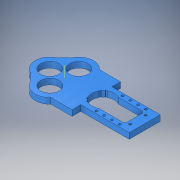
# Autodesk Inventor part: 000.401 - Опорная платформа
Saved by Autodesk Inventor 2019 (Build 230136000, 136)
## iProperties
Created: 2020-03-18
Part Number: 000.401 - Опорная платформа
Material: Пластик АБС
Document SubType Name: Modeling
Designer: Петров Иван
Density: 1.06 g/cm^3
Appearance: Голубой
Author: Петров Иван
Autodesk Inventor part; units mm, degrees
ref_plane "YZ Plane" through (0, 0, 0) normal (1, 0, 0) x (0, 1, 0)
ref_plane "XZ Plane" through (0, 0, 0) normal (0, 1, 0) x (-1, 0, 0)
ref_plane "XY Plane" through (0, 0, 0) normal (0, 0, 1) x (1, 0, 0)
sketch "Эскиз1" plane through (0, 0, 0) normal (0, 1, 0) x (-1, 0, 0)
  circle A0 centre (0, 0) radius 13.8
  circle A1 centre (-8, 0) radius 1.2
  circle A2 centre (0, -8) radius 1.2
  circle A3 centre (8, 0) radius 1.2
  circle A4 centre (0, 8) radius 1.2
  circle A5 centre (-7.7782, 7.7782) radius 1.2813
  circle A6 centre (-11, 0) radius 1.2813
  circle A7 centre (-7.7782, -7.7782) radius 1.2813
  circle A8 centre (0, -11) radius 1.2812
  circle A9 centre (7.7782, -7.7782) radius 1.2812
  circle A10 centre (11, 0) radius 1.2813
  circle A11 centre (7.7782, 7.7782) radius 1.2812
  circle A12 centre (0, 11) radius 1.2812
  circle A13 centre (0, 0) radius 5
  circle A14 centre (0, 0) radius 14
  circle A15 centre (0, 0) radius 1.55
  circle A16 centre (0, 0) radius 1.75
  circle A17 centre (0, 0) radius 25
  dimension "d0" = 50
  constraints: 18 centre point, 1 coincident
  measures "d0" diameter of A17
extrude "Выдавливание1" add sketch "Эскиз1" along normal blind 6 contours A0 | A1 | A2 | A3 | A4 | A5 | A6 | A7 | A8 | A9 | A10 | A11 | A12 | A13 | A14 | A15 | A16 | A17
sketch "Эскиз2" plane through (0, 6, 0) normal (0, 1, 0) x (1, 0, 0)
  line L0 (25, 0) -> (100, 0)
  circle A0 centre (100, 0) radius 25
  line L1 (50, 0) -> (50, -20)
  line L2 (50, 0) -> (50, 20)
  circle A1 centre (0, 0) radius 25 projected
  arc A2 (4.9455, 24.506) -> (95.0545, 24.506) centre (50, 247.5) ccw
  arc A3 (95.0545, -24.506) -> (4.9455, -24.506) centre (50, -247.5) ccw
  line L3 (100, 25) -> (0, 25)
  line L4 (0, -25) -> (100, -25)
  line L5 (50, 20) -> (50, 25)
  line L6 (50, -20) -> (50, -25)
  line L7 (50, 25) -> (50, -25)
  dimension "d3" = 100
  dimension "d4" = 50
  dimension "d5" = 20
  dimension "d6" = 20
  constraints: 16 end point, 15 point on circle, 3 centre point, 3 tangent, 2 midpoint, 2 vertical, 1 coincident, 1 collinear, 1 horizontal, 1 point on line
  measures "d3" distance of point (0, 0) L0.end
  measures "d4" diameter of A0
  measures "d5" distance of L1.start L1.end
  measures "d6" distance of L1.start L2.end
extrude "Выдавливание2" add sketch "Эскиз2" against normal blind 6 contours A1 A2 L2 L0 | L0 L1 A3 A1 | A1 L3 L5 A2 | A3 L6 L4 A1
sketch "Эскиз7" plane through (0, 6, 0) normal (0, 1, 0) x (1, 0, 0)
  line L0 (100, 0) -> (100, 15)
  line L1 (100, 0) -> (100, -15)
  circle A0 centre (100, 15) radius 3
  circle A1 centre (100, -15) radius 3
  line L2 (100, 0) -> (115, 0)
  circle A2 centre (115, 0) radius 3
  point P0 (0, 0)
  dimension "d23" = 15
  dimension "d24" = 15
  dimension "d25" = 6
  dimension "d26" = 6
  dimension "d27" = 15
  dimension "d28" = 6
  constraints: 6 end point, 3 centre point, 3 coincident, 2 vertical, 1 horizontal, 1 other
  measures "d23" distance of L0.start L0.end
  measures "d24" distance of L0.start L1.end
  measures "d25" diameter of A0
  measures "d26" diameter of A1
  measures "d27" distance of L0.start L2.end
  measures "d28" diameter of A2
extrude "Выдавливание7" [suppressed]
move faces "Перенос1" translate (33, 0, 0) faces at (50, 4, 8.3333)
sketch "Эскиз11" plane through (0, 6, 0) normal (0, 1, 0) x (1, 0, 0)
  line L0 (83, -25) -> (0, -25) projected
  line L1 (83, -25) -> (33, -25)
  line L2 (33, -25) -> (33, -16)
  line L3 (33, -16) -> (83, -16)
  line L4 (83, -16) -> (83, -25)
  point P0 (0, 0)
  dimension "d41" = 50
  dimension "d42" = 9
  constraints: 8 end point, 2 parallel, 1 horizontal, 1 perpendicular
  measures "d41" distance of L2.end L3.end
  measures "d42" distance of L1.end L2.end
extrude "Выдавливание11" cut sketch "Эскиз11" against normal blind 10
mirror "Зеркальное отражение2" about plane through (0, 0, 0) normal (0, 0, 1) of "Выдавливание11"
sketch "Эскиз12" plane through (0, 6, 0) normal (0, 1, 0) x (1, 0, 0)
  line L0 (32.95, -10) -> (71.0915, -10)
  line L1 (32.95, -10) -> (32.95, -11.4565)
  arc A0 (32.95, -11.4565) -> (33.5, -11.5) centre (33.5, -8) ccw
  line L2 (33.5, -11.5) -> (42, -11.5)
  line L3 (42, -11.5) -> (42, -13)
  line L4 (42, -13) -> (43.5, -13)
  line L5 (43.5, -13) -> (43.5, -15)
  line L6 (43.5, -15) -> (50, -15)
  line L7 (50, -15) -> (50, -13)
  line L8 (50, -13) -> (51.5, -13)
  line L9 (51.5, -13) -> (51.5, -15)
  line L10 (51.5, -15) -> (58, -15)
  line L11 (58, -15) -> (58, -13)
  line L12 (58, -13) -> (59.5, -13)
  line L13 (59.5, -13) -> (59.5, -15)
  line L14 (59.5, -15) -> (66, -15)
  line L15 (66, -15) -> (66, -13)
  line L16 (66, -13) -> (67.5, -13)
  line L17 (67.5, -13) -> (67.5, -15)
  line L18 (67.5, -15) -> (74, -15)
  line L19 (74, -15) -> (74, -13)
  line L20 (74, -13) -> (75.5, -13)
  line L21 (75.5, -13) -> (75.5, -11.25)
  line L22 (75.5, -11.25) -> (77.5, -11.25)
  line L23 (77.5, -11.25) -> (77.5, -4.75)
  line L24 (77.5, -4.75) -> (75.5, -4.75)
  line L25 (75.5, -4.75) -> (75.5, 4.75)
  line L26 (75.5, 4.75) -> (77.5, 4.75)
  line L27 (77.5, 4.75) -> (77.5, 11.25)
  line L28 (77.5, 11.25) -> (75.5, 11.25)
  line L29 (75.5, 11.25) -> (75.5, 13)
  line L30 (75.5, 13) -> (74, 13)
  line L31 (74, 13) -> (74, 15)
  line L32 (74, 15) -> (67.5, 15)
  line L33 (67.5, 15) -> (67.5, 13)
  line L34 (67.5, 13) -> (66, 13)
  line L35 (66, 13) -> (66, 15)
  line L36 (66, 15) -> (59.5, 15)
  line L37 (59.5, 15) -> (59.5, 13)
  line L38 (59.5, 13) -> (58, 13)
  line L39 (58, 13) -> (58, 15)
  line L40 (58, 15) -> (51.5, 15)
  line L41 (51.5, 15) -> (51.5, 13)
  line L42 (51.5, 13) -> (50, 13)
  line L43 (50, 13) -> (50, 15)
  line L44 (50, 15) -> (43.5, 15)
  line L45 (43.5, 15) -> (43.5, 13)
  line L46 (43.5, 13) -> (42, 13)
  line L47 (42, 13) -> (42, 11.5)
  line L48 (42, 11.5) -> (33.5, 11.5)
  arc A1 (33.5, 11.5) -> (32.9779, 11.4608) centre (33.5, 8) ccw
  line L49 (32.9779, 11.4608) -> (32.9779, 10)
  line L50 (71.0279, 10) -> (32.9779, 10)
  line L51 (71.0279, 10) -> (71.1016, 9.9543)
  arc A2 (72.4429, 8.5313) -> (71.1016, 9.9543) centre (73, 10.4) ccw
  line L52 (72.4429, 8.5313) -> (72.5, 8.4256)
  line L53 (72.5, -8.5152) -> (72.5, 8.4256)
  arc A3 (71.0915, -10) -> (72.5, -8.5152) centre (73, -10.4) ccw
  circle A4 centre (54.75, -13.5) radius 1.25
  circle A5 centre (70.75, -13.5) radius 1.25
  circle A6 centre (76, 8) radius 1.25
  circle A7 centre (70.75, 13.5) radius 1.25
  circle A8 centre (62.75, 13.5) radius 1.25
  circle A9 centre (54.75, 13.5) radius 1.25
  circle A10 centre (46.75, 13.5) radius 1.25
  circle A11 centre (76, -8) radius 1.25
  circle A12 centre (62.75, -13.5) radius 1.25
  circle A13 centre (46.75, -13.5) radius 1.25
  arc A14 (32.95, -9.25) -> (31, -7.3) centre (31, -9.25) ccw
  line L54 (32.95, -9.25) -> (32.95, -10)
  line L55 (32.95, -10) -> (48.95, -10)
  line L56 (48.95, -10) -> (48.75, -9.8)
  line L57 (48.75, -7.0711) -> (48.75, -9.8)
  arc A15 (48.75, -7.0711) -> (48.75, 7.0711) centre (40, 0) ccw
  line L58 (48.75, 9.8) -> (48.75, 7.0711)
  line L59 (48.75, 9.8) -> (48.95, 10)
  line L60 (48.95, 10) -> (32.95, 10)
  line L61 (32.95, 10) -> (32.95, 9.25)
  arc A16 (31, 7.3) -> (32.95, 9.25) centre (31, 9.25) ccw
  line L62 (31, 7.3) -> (30, 7.3)
  line L63 (30, 7.3) -> (30, -7.3)
  line L64 (30, -7.3) -> (31, -7.3)
  circle A17 centre (40, 0) radius 9.1
  line L65 (48.95, 10) -> (32.95, 10)
  line L66 (42, 13) -> (42, 11.5)
  line L67 (33.5, 13) -> (42, 13)
  line L68 (33.5, 11.5) -> (33.5, 13)
  line L69 (42, 11.5) -> (33.5, 11.5)
  arc A18 (33.5, 13) -> (32.9501, 12.9697) centre (33.5, 8) ccw
  spline S0 degree 3 poles (32.9501, 12.9697) (32.9501, 12.9689) (32.9503, 12.9605) (32.9503, 12.9597) (32.9503, 12.959) (32.9503, 12.9582) (32.9503, 12.9574) (32.9503, 12.9541) (32.9504, 12.9501) (32.9505, 12.9454) (32.9505, 12.9438) (32.9505, 12.9421) (32.9505, 12.9403) (32.9505, 12.9395) (32.9506, 12.9387) (32.9506, 12.9379) (32.9506, 12.9353) (32.9506, 12.9324) (32.9507, 12.9294) (32.9508, 12.9234) (32.9509, 12.9168) (32.951, 12.9095) (32.951, 12.9077) (32.951, 12.9059) (32.951, 12.9041) (32.9511, 12.8983) (32.9512, 12.8922) (32.9513, 12.8858) (32.9514, 12.8786) (32.9515, 12.8711) (32.9516, 12.8629) (32.9516, 12.8601) (32.9517, 12.8571) (32.9517, 12.8541) (32.9519, 12.8456) (32.952, 12.8366) (32.9521, 12.8272) (32.9523, 12.8162) (32.9524, 12.8046) (32.9526, 12.7924) (32.9528, 12.7801) (32.953, 12.7673) (32.9532, 12.7538) (32.9533, 12.7471) (32.9534, 12.7401) (32.9535, 12.7331) (32.9536, 12.7264) (32.9537, 12.7196) (32.9538, 12.7126) (32.954, 12.6978) (32.9542, 12.6823) (32.9545, 12.6664) (32.9547, 12.6528) (32.9549, 12.6387) (32.9551, 12.6244) (32.9553, 12.6118) (32.9555, 12.5991) (32.9557, 12.5862) (32.9558, 12.5798) (32.9559, 12.5734) (32.956, 12.5669) (32.9562, 12.5538) (32.9564, 12.5402) (32.9567, 12.5259) (32.957, 12.5031) (32.9574, 12.4796) (32.9578, 12.4556) (32.958, 12.4458) (32.9581, 12.4359) (32.9583, 12.4258) (32.9585, 12.4158) (32.9586, 12.4056) (32.9588, 12.3954) (32.9592, 12.3748) (32.9595, 12.354) (32.9599, 12.3329) (32.9601, 12.3203) (32.9603, 12.3076) (32.9605, 12.2948) (32.9607, 12.286) (32.9608, 12.2773) (32.961, 12.2685) (32.9614, 12.2466) (32.9618, 12.2245) (32.9622, 12.2021) (32.9624, 12.1909) (32.9626, 12.1796) (32.9628, 12.1683) (32.963, 12.1568) (32.9632, 12.1454) (32.9634, 12.1339) (32.9638, 12.1145) (32.9642, 12.0951) (32.9645, 12.0752) (32.9646, 12.0714) (32.9647, 12.0676) (32.9648, 12.0637) (32.9649, 12.0547) (32.9651, 12.0456) (32.9653, 12.0365) (32.9656, 12.0216) (32.9659, 12.0067) (32.9662, 11.9916) (32.9666, 11.9672) (32.9671, 11.9425) (32.9676, 11.9178) (32.9681, 11.8931) (32.9687, 11.8682) (32.9692, 11.8433) (32.9697, 11.8183) (32.9702, 11.7932) (32.9708, 11.7681) (32.9719, 11.7177) (32.973, 11.6669) (32.9742, 11.6157) (32.9754, 11.5645) (32.9766, 11.5128) (32.9779, 11.4608) knots 0.064201 0.064201 0.064201 0.064201 0.072529 0.072529 0.072529 0.080597 0.080597 0.080597 0.113423 0.113423 0.113423 0.125 0.125 0.125 0.12994 0.12994 0.12994 0.146482 0.146482 0.146482 0.17952 0.17952 0.17952 0.1875 0.1875 0.1875 0.212571 0.212571 0.212571 0.240274 0.240274 0.240274 0.25 0.25 0.25 0.277642 0.277642 0.277642 0.310147 0.310147 0.310147 0.342874 0.342874 0.342874 0.3593 0.3593 0.3593 0.375 0.375 0.375 0.408683 0.408683 0.408683 0.4375 0.4375 0.4375 0.462715 0.462715 0.462715 0.475013 0.475013 0.475013 0.5 0.5 0.5 0.540067 0.540067 0.540067 0.556372 0.556372 0.556372 0.572723 0.572723 0.572723 0.605497 0.605497 0.605497 0.625 0.625 0.625 0.638264 0.638264 0.638264 0.671081 0.671081 0.671081 0.6875 0.6875 0.6875 0.704131 0.704131 0.704131 0.732078 0.732078 0.732078 0.737463 0.737463 0.737463 0.75 0.75 0.75 0.770238 0.770238 0.770238 0.802948 0.802948 0.802948 0.835688 0.835688 0.835688 0.868461 0.868461 0.868461 0.93413 0.93413 0.93413 1 1 1 1
  arc A19 (33.5, 11.5) -> (32.9779, 11.4608) centre (33.5, 8) ccw
  line L70 (33.5, 11.5) -> (33.5, 13)
  arc A20 (32.9501, 12.9697) -> (28.5, 8) centre (33.5, 8) ccw
  line L71 (28.5, 7.3) -> (28.5, 8)
  line L72 (28.5, -7.3) -> (28.5, 7.3)
  line L73 (28.5, -8) -> (28.5, -7.3)
  arc A21 (28.5, -8) -> (32.9271, -12.9671) centre (33.5, -8) ccw
  line L74 (42, -13) -> (33.5, -13)
  arc A22 (32.9271, -12.9671) -> (33.5, -13) centre (33.5, -8) ccw
  line L75 (43.5, -16) -> (43.5, -15)
  line L76 (50, -16) -> (43.5, -16)
  line L77 (50, -15) -> (50, -16)
  line L78 (43.5, -15) -> (50, -15)
  line L79 (51.5, -16) -> (51.5, -15)
  line L80 (58, -16) -> (51.5, -16)
  line L81 (58, -15) -> (58, -16)
  line L82 (51.5, -15) -> (58, -15)
  line L83 (59.5, -16) -> (59.5, -15)
  line L84 (66, -16) -> (59.5, -16)
  line L85 (66, -15) -> (66, -16)
  line L86 (59.5, -15) -> (66, -15)
  line L87 (67.5, -16) -> (67.5, -15)
  line L88 (74, -16) -> (67.5, -16)
  line L89 (74, -15) -> (74, -16)
  line L90 (67.5, -15) -> (74, -15)
  line L91 (78.5, -11.25) -> (77.5, -11.25)
  line L92 (78.5, -4.75) -> (78.5, -11.25)
  line L93 (77.5, -4.75) -> (78.5, -4.75)
  line L94 (77.5, -11.25) -> (77.5, -4.75)
  line L95 (78.5, 4.75) -> (77.5, 4.75)
  line L96 (78.5, 11.25) -> (78.5, 4.75)
  line L97 (77.5, 11.25) -> (78.5, 11.25)
  line L98 (77.5, 4.75) -> (77.5, 11.25)
  line L99 (74, 16) -> (74, 15)
  line L100 (67.5, 16) -> (74, 16)
  line L101 (67.5, 15) -> (67.5, 16)
  line L102 (74, 15) -> (67.5, 15)
  line L103 (66, 16) -> (66, 15)
  line L104 (59.5, 16) -> (66, 16)
  line L105 (59.5, 15) -> (59.5, 16)
  line L106 (66, 15) -> (59.5, 15)
  line L107 (51.5, 16) -> (58, 16)
  line L108 (58, 16) -> (58, 15)
  line L109 (51.5, 16) -> (58, 16)
  line L110 (51.5, 15) -> (51.5, 16)
  line L111 (58, 15) -> (51.5, 15)
  line L112 (50, 16) -> (50, 15)
  line L113 (43.5, 16) -> (50, 16)
  line L114 (43.5, 15) -> (43.5, 16)
  line L115 (50, 15) -> (43.5, 15)
  spline S1 degree 3 poles (32.95, -11.4565) (32.9497, -11.4689) (32.9495, -11.4813) (32.9492, -11.4937) (32.9487, -11.5195) (32.9482, -11.5454) (32.9477, -11.5712) (32.9472, -11.5969) (32.9467, -11.6225) (32.9462, -11.6481) (32.9456, -11.6821) (32.9449, -11.716) (32.9443, -11.7496) (32.944, -11.7664) (32.9437, -11.7832) (32.9434, -11.7999) (32.943, -11.825) (32.9425, -11.85) (32.9421, -11.8749) (32.942, -11.8808) (32.9419, -11.8868) (32.9418, -11.8927) (32.9415, -11.9115) (32.9412, -11.9304) (32.9409, -11.9492) (32.9407, -11.9616) (32.9405, -11.9739) (32.9403, -11.986) (32.9401, -11.9983) (32.9399, -12.0104) (32.9397, -12.0224) (32.9396, -12.0258) (32.9396, -12.0292) (32.9395, -12.0327) (32.9392, -12.0531) (32.9389, -12.0734) (32.9386, -12.0936) (32.9379, -12.1324) (32.9374, -12.1706) (32.9368, -12.208) (32.9367, -12.2155) (32.9366, -12.2229) (32.9365, -12.2303) (32.9362, -12.2507) (32.9359, -12.2709) (32.9356, -12.2908) (32.9353, -12.3141) (32.935, -12.3369) (32.9346, -12.3594) (32.9345, -12.3699) (32.9343, -12.3802) (32.9342, -12.3905) (32.9341, -12.3973) (32.934, -12.4041) (32.9339, -12.4108) (32.9339, -12.4142) (32.9338, -12.4176) (32.9338, -12.421) (32.9336, -12.4356) (32.9334, -12.4501) (32.9332, -12.4643) (32.9331, -12.4696) (32.9331, -12.4747) (32.933, -12.4799) (32.9328, -12.4947) (32.9326, -12.509) (32.9324, -12.5227) (32.9324, -12.527) (32.9323, -12.5314) (32.9323, -12.5357) (32.932, -12.5537) (32.9318, -12.5714) (32.9316, -12.5885) (32.9314, -12.6056) (32.9312, -12.6223) (32.931, -12.6384) (32.9308, -12.6545) (32.9306, -12.6702) (32.9304, -12.6853) (32.9303, -12.6935) (32.9302, -12.7016) (32.9301, -12.7095) (32.93, -12.7161) (32.9299, -12.7227) (32.9298, -12.7291) (32.9298, -12.7362) (32.9297, -12.7431) (32.9296, -12.7499) (32.9295, -12.7567) (32.9294, -12.7633) (32.9293, -12.7697) (32.9293, -12.7755) (32.9292, -12.7811) (32.9291, -12.7866) (32.9291, -12.7934) (32.929, -12.8001) (32.9289, -12.8066) (32.9288, -12.8161) (32.9287, -12.8252) (32.9286, -12.8338) (32.9286, -12.8358) (32.9286, -12.8378) (32.9285, -12.8397) (32.9285, -12.8437) (32.9284, -12.8476) (32.9284, -12.8514) (32.9282, -12.8675) (32.928, -12.8819) (32.9279, -12.8948) (32.9278, -12.9027) (32.9277, -12.9101) (32.9276, -12.9167) (32.9276, -12.9234) (32.9275, -12.9295) (32.9274, -12.9349) (32.9274, -12.9403) (32.9273, -12.945) (32.9273, -12.949) (32.9272, -12.953) (32.9272, -12.9564) (32.9272, -12.9591) (32.9271, -12.9644) (32.9271, -12.9671) (32.9271, -12.9671) knots 0 0 0 0 0.015717 0.015717 0.015717 0.048574 0.048574 0.048574 0.081322 0.081322 0.081322 0.125 0.125 0.125 0.146869 0.146869 0.146869 0.179663 0.179663 0.179663 0.1875 0.1875 0.1875 0.212348 0.212348 0.212348 0.228682 0.228682 0.228682 0.245216 0.245216 0.245216 0.25 0.25 0.25 0.278672 0.278672 0.278672 0.333784 0.333784 0.333784 0.344755 0.344755 0.344755 0.375 0.375 0.375 0.410279 0.410279 0.410279 0.42665 0.42665 0.42665 0.4375 0.4375 0.4375 0.443003 0.443003 0.443003 0.466515 0.466515 0.466515 0.475131 0.475131 0.475131 0.5 0.5 0.5 0.507943 0.507943 0.507943 0.541148 0.541148 0.541148 0.574177 0.574177 0.574177 0.607119 0.607119 0.607119 0.625 0.625 0.625 0.640065 0.640065 0.640065 0.65654 0.65654 0.65654 0.672965 0.672965 0.672965 0.6875 0.6875 0.6875 0.705429 0.705429 0.705429 0.731487 0.731487 0.731487 0.737562 0.737562 0.737562 0.75 0.75 0.75 0.803346 0.803346 0.803346 0.83629 0.83629 0.83629 0.869201 0.869201 0.869201 0.902051 0.902051 0.902051 0.934818 0.934818 0.934818 1 1 1 1
  line L116 (32.75, -12.7684) -> (32.75, -11.4565)
  line L117 (32.75, -11.4565) -> (32.75, -10)
  line L118 (32.95, -10) -> (32.75, -10)
  line L119 (32.95, -11.4565) -> (32.75, -11.4565)
  line L120 (32.75, -12.7684) -> (32.75, -11.4565)
  line L121 (32.9271, -12.9671) -> (32.75, -12.7684)
  spline S2 degree 3 poles (32.95, -11.4565) (32.9497, -11.4689) (32.9495, -11.4813) (32.9492, -11.4937) (32.9487, -11.5195) (32.9482, -11.5454) (32.9477, -11.5712) (32.9472, -11.5969) (32.9467, -11.6225) (32.9462, -11.6481) (32.9456, -11.6821) (32.9449, -11.716) (32.9443, -11.7496) (32.944, -11.7664) (32.9437, -11.7832) (32.9434, -11.7999) (32.943, -11.825) (32.9425, -11.85) (32.9421, -11.8749) (32.942, -11.8808) (32.9419, -11.8868) (32.9418, -11.8927) (32.9415, -11.9115) (32.9412, -11.9304) (32.9409, -11.9492) (32.9407, -11.9616) (32.9405, -11.9739) (32.9403, -11.986) (32.9401, -11.9983) (32.9399, -12.0104) (32.9397, -12.0224) (32.9396, -12.0258) (32.9396, -12.0292) (32.9395, -12.0327) (32.9392, -12.0531) (32.9389, -12.0734) (32.9386, -12.0936) (32.938, -12.1324) (32.9374, -12.1706) (32.9368, -12.208) (32.9367, -12.2155) (32.9366, -12.2229) (32.9365, -12.2303) (32.9362, -12.2507) (32.9359, -12.2709) (32.9356, -12.2908) (32.9353, -12.3141) (32.935, -12.3369) (32.9346, -12.3594) (32.9345, -12.3699) (32.9344, -12.3802) (32.9342, -12.3905) (32.9341, -12.3973) (32.934, -12.4041) (32.9339, -12.4108) (32.9339, -12.4142) (32.9338, -12.4176) (32.9338, -12.421) (32.9336, -12.4356) (32.9334, -12.4501) (32.9332, -12.4643) (32.9331, -12.4696) (32.9331, -12.4747) (32.933, -12.4799) (32.9328, -12.4947) (32.9326, -12.509) (32.9324, -12.5227) (32.9324, -12.527) (32.9323, -12.5314) (32.9323, -12.5357) (32.932, -12.5537) (32.9318, -12.5714) (32.9316, -12.5885) (32.9314, -12.6056) (32.9312, -12.6223) (32.931, -12.6384) (32.9308, -12.6545) (32.9306, -12.6702) (32.9304, -12.6853) (32.9303, -12.6935) (32.9302, -12.7016) (32.9301, -12.7095) (32.93, -12.7161) (32.9299, -12.7227) (32.9298, -12.7291) (32.9298, -12.7362) (32.9297, -12.7431) (32.9296, -12.7499) (32.9295, -12.7567) (32.9294, -12.7633) (32.9294, -12.7697) (32.9293, -12.7755) (32.9292, -12.7811) (32.9292, -12.7866) (32.9291, -12.7934) (32.929, -12.8001) (32.9289, -12.8066) (32.9288, -12.8161) (32.9287, -12.8252) (32.9286, -12.8338) (32.9286, -12.8358) (32.9286, -12.8378) (32.9285, -12.8397) (32.9285, -12.8437) (32.9284, -12.8476) (32.9284, -12.8514) (32.9282, -12.8675) (32.928, -12.8819) (32.9279, -12.8948) (32.9278, -12.9027) (32.9277, -12.9101) (32.9277, -12.9167) (32.9276, -12.9234) (32.9275, -12.9295) (32.9274, -12.9349) (32.9274, -12.9403) (32.9273, -12.945) (32.9273, -12.949) (32.9272, -12.953) (32.9272, -12.9564) (32.9272, -12.9591) (32.9271, -12.9644) (32.9271, -12.9671) (32.9271, -12.9671) knots 0 0 0 0 0.015717 0.015717 0.015717 0.048574 0.048574 0.048574 0.081322 0.081322 0.081322 0.125 0.125 0.125 0.146869 0.146869 0.146869 0.179663 0.179663 0.179663 0.1875 0.1875 0.1875 0.212348 0.212348 0.212348 0.228682 0.228682 0.228682 0.245216 0.245216 0.245216 0.25 0.25 0.25 0.278672 0.278672 0.278672 0.333784 0.333784 0.333784 0.344755 0.344755 0.344755 0.375 0.375 0.375 0.410279 0.410279 0.410279 0.42665 0.42665 0.42665 0.4375 0.4375 0.4375 0.443003 0.443003 0.443003 0.466515 0.466515 0.466515 0.475131 0.475131 0.475131 0.5 0.5 0.5 0.507943 0.507943 0.507943 0.541148 0.541148 0.541148 0.574177 0.574177 0.574177 0.607119 0.607119 0.607119 0.625 0.625 0.625 0.640065 0.640065 0.640065 0.65654 0.65654 0.65654 0.672965 0.672965 0.672965 0.6875 0.6875 0.6875 0.705429 0.705429 0.705429 0.731487 0.731487 0.731487 0.737562 0.737562 0.737562 0.75 0.75 0.75 0.803346 0.803346 0.803346 0.83629 0.83629 0.83629 0.869201 0.869201 0.869201 0.902051 0.902051 0.902051 0.934818 0.934818 0.934818 1 1 1 1
  line L122 (32.75, -10) -> (32.95, -10)
  line L123 (32.75, -11.4565) -> (32.75, -10)
  line L124 (32.95, -11.4565) -> (32.75, -11.4565)
  line L125 (32.95, -10) -> (32.95, -11.4565)
  line L126 (32.75, 11.4608) -> (32.9779, 11.4608)
  spline S3 degree 3 poles (32.9501, 12.9697) (32.9501, 12.9689) (32.9503, 12.9605) (32.9503, 12.9597) (32.9503, 12.959) (32.9503, 12.9582) (32.9503, 12.9574) (32.9503, 12.9541) (32.9504, 12.9501) (32.9505, 12.9454) (32.9505, 12.9438) (32.9505, 12.9421) (32.9505, 12.9403) (32.9505, 12.9395) (32.9506, 12.9387) (32.9506, 12.9379) (32.9506, 12.9353) (32.9506, 12.9324) (32.9507, 12.9294) (32.9508, 12.9234) (32.9509, 12.9168) (32.951, 12.9095) (32.951, 12.9077) (32.951, 12.9059) (32.951, 12.9041) (32.9511, 12.8983) (32.9512, 12.8922) (32.9513, 12.8858) (32.9514, 12.8786) (32.9515, 12.8711) (32.9516, 12.8629) (32.9516, 12.8601) (32.9517, 12.8571) (32.9517, 12.8541) (32.9519, 12.8456) (32.952, 12.8366) (32.9521, 12.8272) (32.9523, 12.8162) (32.9524, 12.8046) (32.9526, 12.7924) (32.9528, 12.7801) (32.953, 12.7673) (32.9532, 12.7538) (32.9533, 12.7471) (32.9534, 12.7401) (32.9535, 12.7331) (32.9536, 12.7264) (32.9537, 12.7196) (32.9538, 12.7126) (32.954, 12.6978) (32.9542, 12.6823) (32.9545, 12.6664) (32.9547, 12.6528) (32.9549, 12.6387) (32.9551, 12.6244) (32.9553, 12.6118) (32.9555, 12.5991) (32.9557, 12.5862) (32.9558, 12.5798) (32.9559, 12.5734) (32.956, 12.5669) (32.9562, 12.5538) (32.9564, 12.5402) (32.9567, 12.5259) (32.957, 12.5031) (32.9574, 12.4796) (32.9578, 12.4556) (32.958, 12.4458) (32.9581, 12.4359) (32.9583, 12.4258) (32.9585, 12.4158) (32.9586, 12.4056) (32.9588, 12.3954) (32.9591, 12.3748) (32.9595, 12.354) (32.9599, 12.3329) (32.9601, 12.3203) (32.9603, 12.3076) (32.9605, 12.2948) (32.9607, 12.286) (32.9608, 12.2773) (32.961, 12.2685) (32.9614, 12.2466) (32.9618, 12.2245) (32.9622, 12.2021) (32.9624, 12.1909) (32.9626, 12.1796) (32.9628, 12.1683) (32.963, 12.1568) (32.9632, 12.1454) (32.9634, 12.1339) (32.9638, 12.1145) (32.9642, 12.0951) (32.9645, 12.0752) (32.9646, 12.0714) (32.9647, 12.0676) (32.9648, 12.0637) (32.9649, 12.0547) (32.9651, 12.0456) (32.9653, 12.0365) (32.9656, 12.0216) (32.9659, 12.0067) (32.9662, 11.9916) (32.9666, 11.9672) (32.9671, 11.9425) (32.9676, 11.9178) (32.9681, 11.8931) (32.9686, 11.8682) (32.9692, 11.8433) (32.9697, 11.8183) (32.9702, 11.7932) (32.9708, 11.7681) (32.9719, 11.7177) (32.973, 11.6669) (32.9742, 11.6157) (32.9754, 11.5645) (32.9766, 11.5128) (32.9779, 11.4608) knots 0.064201 0.064201 0.064201 0.064201 0.072529 0.072529 0.072529 0.080597 0.080597 0.080597 0.113423 0.113423 0.113423 0.125 0.125 0.125 0.12994 0.12994 0.12994 0.146482 0.146482 0.146482 0.17952 0.17952 0.17952 0.1875 0.1875 0.1875 0.212571 0.212571 0.212571 0.240274 0.240274 0.240274 0.25 0.25 0.25 0.277642 0.277642 0.277642 0.310147 0.310147 0.310147 0.342874 0.342874 0.342874 0.3593 0.3593 0.3593 0.375 0.375 0.375 0.408683 0.408683 0.408683 0.4375 0.4375 0.4375 0.462715 0.462715 0.462715 0.475013 0.475013 0.475013 0.5 0.5 0.5 0.540067 0.540067 0.540067 0.556372 0.556372 0.556372 0.572723 0.572723 0.572723 0.605497 0.605497 0.605497 0.625 0.625 0.625 0.638264 0.638264 0.638264 0.671081 0.671081 0.671081 0.6875 0.6875 0.6875 0.704131 0.704131 0.704131 0.732078 0.732078 0.732078 0.737463 0.737463 0.737463 0.75 0.75 0.75 0.770238 0.770238 0.770238 0.802948 0.802948 0.802948 0.835688 0.835688 0.835688 0.868461 0.868461 0.868461 0.93413 0.93413 0.93413 1 1 1 1
  line L127 (32.7706, 12.7443) -> (32.9501, 12.9697)
  line L128 (32.75, 12.7184) -> (32.7706, 12.7443)
  line L129 (32.75, 11.4608) -> (32.75, 12.7184)
  line L130 (32.9779, 10) -> (32.75, 10)
  line L131 (32.9779, 11.4608) -> (32.9779, 10)
  line L132 (32.75, 11.4608) -> (32.9779, 11.4608)
  line L133 (32.75, 10) -> (32.75, 11.4608)
  arc A23 (32.95, -11.4565) -> (33.5, -11.5) centre (33.5, -8) ccw
  spline S4 degree 3 poles (32.95, -11.4565) (32.9497, -11.4689) (32.9495, -11.4813) (32.9492, -11.4937) (32.9487, -11.5195) (32.9482, -11.5454) (32.9477, -11.5712) (32.9472, -11.5969) (32.9467, -11.6225) (32.9462, -11.6481) (32.9456, -11.6821) (32.9449, -11.716) (32.9443, -11.7496) (32.944, -11.7664) (32.9437, -11.7832) (32.9434, -11.7999) (32.943, -11.825) (32.9425, -11.85) (32.9421, -11.8749) (32.942, -11.8808) (32.9419, -11.8868) (32.9418, -11.8927) (32.9415, -11.9115) (32.9412, -11.9304) (32.9409, -11.9492) (32.9407, -11.9616) (32.9405, -11.9739) (32.9403, -11.986) (32.9401, -11.9983) (32.9399, -12.0104) (32.9397, -12.0224) (32.9396, -12.0258) (32.9396, -12.0292) (32.9395, -12.0327) (32.9392, -12.0531) (32.9389, -12.0734) (32.9386, -12.0936) (32.938, -12.1324) (32.9374, -12.1706) (32.9368, -12.208) (32.9367, -12.2155) (32.9366, -12.2229) (32.9365, -12.2303) (32.9362, -12.2507) (32.9359, -12.2709) (32.9356, -12.2908) (32.9353, -12.3141) (32.935, -12.3369) (32.9346, -12.3594) (32.9345, -12.3699) (32.9344, -12.3802) (32.9342, -12.3905) (32.9341, -12.3973) (32.934, -12.4041) (32.9339, -12.4108) (32.9339, -12.4142) (32.9338, -12.4176) (32.9338, -12.421) (32.9336, -12.4356) (32.9334, -12.4501) (32.9332, -12.4643) (32.9331, -12.4696) (32.9331, -12.4747) (32.933, -12.4799) (32.9328, -12.4947) (32.9326, -12.509) (32.9324, -12.5227) (32.9324, -12.527) (32.9323, -12.5314) (32.9323, -12.5357) (32.932, -12.5537) (32.9318, -12.5714) (32.9316, -12.5885) (32.9314, -12.6056) (32.9312, -12.6223) (32.931, -12.6384) (32.9308, -12.6545) (32.9306, -12.6702) (32.9304, -12.6853) (32.9303, -12.6935) (32.9302, -12.7016) (32.9301, -12.7095) (32.93, -12.7161) (32.9299, -12.7227) (32.9298, -12.7291) (32.9298, -12.7362) (32.9297, -12.7431) (32.9296, -12.7499) (32.9295, -12.7567) (32.9294, -12.7633) (32.9294, -12.7697) (32.9293, -12.7755) (32.9292, -12.7811) (32.9292, -12.7866) (32.9291, -12.7934) (32.929, -12.8001) (32.9289, -12.8066) (32.9288, -12.8161) (32.9287, -12.8252) (32.9286, -12.8338) (32.9286, -12.8358) (32.9286, -12.8378) (32.9285, -12.8397) (32.9285, -12.8437) (32.9284, -12.8476) (32.9284, -12.8514) (32.9282, -12.8675) (32.928, -12.8819) (32.9279, -12.8948) (32.9278, -12.9027) (32.9277, -12.9101) (32.9277, -12.9167) (32.9276, -12.9234) (32.9275, -12.9295) (32.9274, -12.9349) (32.9274, -12.9403) (32.9273, -12.945) (32.9273, -12.949) (32.9272, -12.953) (32.9272, -12.9564) (32.9272, -12.9591) (32.9271, -12.9644) (32.9271, -12.9671) (32.9271, -12.9671) knots 0 0 0 0 0.015717 0.015717 0.015717 0.048574 0.048574 0.048574 0.081322 0.081322 0.081322 0.125 0.125 0.125 0.146869 0.146869 0.146869 0.179663 0.179663 0.179663 0.1875 0.1875 0.1875 0.212348 0.212348 0.212348 0.228682 0.228682 0.228682 0.245216 0.245216 0.245216 0.25 0.25 0.25 0.278672 0.278672 0.278672 0.333784 0.333784 0.333784 0.344755 0.344755 0.344755 0.375 0.375 0.375 0.410279 0.410279 0.410279 0.42665 0.42665 0.42665 0.4375 0.4375 0.4375 0.443003 0.443003 0.443003 0.466515 0.466515 0.466515 0.475131 0.475131 0.475131 0.5 0.5 0.5 0.507943 0.507943 0.507943 0.541148 0.541148 0.541148 0.574177 0.574177 0.574177 0.607119 0.607119 0.607119 0.625 0.625 0.625 0.640065 0.640065 0.640065 0.65654 0.65654 0.65654 0.672965 0.672965 0.672965 0.6875 0.6875 0.6875 0.705429 0.705429 0.705429 0.731487 0.731487 0.731487 0.737562 0.737562 0.737562 0.75 0.75 0.75 0.803346 0.803346 0.803346 0.83629 0.83629 0.83629 0.869201 0.869201 0.869201 0.902051 0.902051 0.902051 0.934818 0.934818 0.934818 1 1 1 1
  arc A24 (32.9271, -12.9671) -> (33.5, -13) centre (33.5, -8) ccw
  line L134 (33.5, -13) -> (33.5, -11.5)
  line L135 (78.5, 4.75) -> (78.5, -4.75)
  circle A25 centre (73, 10.4) radius 1.95
  circle A26 centre (73, -10.4) radius 1.95
  line L136 (83, -16) -> (83, 16) projected
  circle A27 centre (40, 0) radius 11.5
  point P0 (40, 0)
  point P1 (28.5, 0)
  point P2 (28.5, 0)
  point P3 (78.5, 0)
  point P4 (83, 0)
  constraints: 272 end point, 28 point on circle, 26 centre point, 3 midpoint, 2 coincident, 1 point on line, 1 tangent, 16 other
extrude "Выдавливание13" cut sketch "Эскиз12" against normal blind 10 contours L56 L57 A27 L58 L59 L50 L51 A25 L52 L53 A26 L0 | L0 A27 L57 L56 | A27 L0 | L0 A27 A14 L63 A16 L50 L58 A15 L57 | L0 L54 A14 A27 | L57 A15 L58 A27 | A27 A14 | A14 L64 L63 A27 | A27 L50 L59 L58 | A27 L63 | L50 A27 | L63 L62 A16 A27 | A27 A16 L61 L60 L50 | A27 A16 | A4 | A5 | A6 | A7 | A8 | A9 | A10 | A11 | A12 | A13 | A17
sketch "Эскиз13" plane through (0, 6, 0) normal (0, 1, 0) x (1, 0, 0)
  circle A0 centre (-14.1421, -14.1421) radius 2.1
  circle A1 centre (10, 0) radius 2.1
  circle A2 centre (-14.1421, 14.1421) radius 2.1
  circle A3 centre (-15.0247, 0.005) radius 9.5
  circle A4 centre (-0.0247, 15.005) radius 9.5
  circle A5 centre (-0.0247, -14.995) radius 9.5
  line L0 (13.7779, -24.9956) -> (13.7779, 25.0044)
  line L1 (13.7779, 25.0044) -> (-0.0275, 25.0044)
  arc A6 (-0.0275, 25.0044) -> (-0.0275, -24.9956) centre (-0.0275, 0.0044) ccw
  line L2 (-0.0275, -24.9956) -> (13.7779, -24.9956)
  point P0 (0, 0)
  point P1 (0, 0)
  constraints: 7 centre point, 6 end point, 2 point on circle
extrude "Выдавливание14" cut sketch "Эскиз13" against normal blind 10 contours A3 | A4 | A5
sketch "Эскиз14" plane through (0, 6, 0) normal (0, 1, 0) x (1, 0, 0)
  circle A0 centre (-0.0247, 15.005) radius 9.5 projected
  arc A1 (-5.585, 1.0736) -> (-13.956, 9.4447) centre (-0.0247, 15.005) ccw
  circle A2 centre (-0.0247, -14.995) radius 9.5 projected
  arc A3 (-13.9504, -9.4341) -> (-5.5856, -1.0692) centre (-0.0247, -14.995) ccw
  circle A4 centre (-15.0247, 0.005) radius 9.5 projected
  arc A5 (-9.4675, 13.9642) -> (-9.4675, -13.9542) centre (-15.0247, 0.005) ccw
  arc A6 (-1.0655, -5.5522) -> (-1.0655, 5.5622) centre (-15.0247, 0.005) ccw
  point P0 (0, 0)
  dimension "d52" = 30
  constraints: 18 point on circle, 4 centre point, 3 coincident
  measures "d52" diameter of A1
extrude "Выдавливание15" add sketch "Эскиз14" against normal blind 6 contours A0 A5 A1 A6 | A0 A6 A1 A4 A5 | A1 A4 A3 A5 | A6 A3 A4 A1 | A5 A2 A6 A3 | A3 A4 A6 A2 A5
equation "\"d6\" = d5"
equation "\"d24\" = d23"
equation "\"d26\" = d25"
equation "\"d27\" = d23"
equation "\"d28\" = d25"
